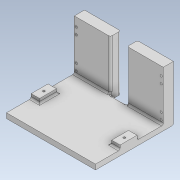
# Autodesk Inventor part: electrical_system_fix_board
Saved by Autodesk Inventor 2020 (Build 240168000, 168)
## iProperties
Created: 2021-01-08
Part Number: electrical_system_fix_board
Material: Generic
Document SubType Name: Modeling
Designer: DELL
Density: 1 g/cm^3
Appearance: Default
Author: DELL
Autodesk Inventor part; units mm, degrees
ref_plane "YZ Plane" through (0, 0, 0) normal (1, 0, 0) x (0, 1, 0)
ref_plane "XZ Plane" through (0, 0, 0) normal (0, 1, 0) x (-1, 0, 0)
ref_plane "XY Plane" through (0, 0, 0) normal (0, 0, 1) x (1, 0, 0)
sketch "Sketch1" plane through (0, 0, 0) normal (0, 0, 1) x (1, 0, 0)
  line L0 (52.5, 32.5) -> (-52.5, 32.5)
  line L1 (-52.5, 32.5) -> (-52.5, -32.5)
  line L2 (-52.5, -32.5) -> (52.5, -32.5)
  line L3 (52.5, -32.5) -> (52.5, 32.5)
  line L4 (52.5, 32.5) -> (-52.5, -32.5) construction
  line L5 (-52.5, 32.5) -> (52.5, -32.5) construction
  line L6 (-10, -32.5) -> (-52.5, -32.5)
  line L7 (-52.5, -32.5) -> (-52.5, 32.5)
  line L8 (-52.5, 32.5) -> (-10, 32.5)
  line L9 (-10, 32.5) -> (-10, -32.5)
  line L10 (-10, -32.5) -> (-52.5, 32.5) construction
  line L11 (-52.5, -32.5) -> (-10, 32.5) construction
  line L12 (10, -32.5) -> (52.5, -32.5)
  line L13 (52.5, -32.5) -> (52.5, 32.5)
  line L14 (52.5, 32.5) -> (10, 32.5)
  line L15 (10, 32.5) -> (10, -32.5)
  line L16 (10, -32.5) -> (52.5, 32.5) construction
  line L17 (52.5, -32.5) -> (10, 32.5) construction
  line L18 (0, 32.5) -> (0, -32.5) construction
  point P0 (0, 0)
  point P1 (-31.25, 0)
  point P2 (31.25, 0)
  point P3 (10, 32.5)
  point P4 (10, -32.5)
  point P5 (-10, 32.5)
  dimension "d0" = 105
  dimension "d1" = 65
  dimension "d2" = 20
  constraints: 38 end point, 8 midpoint, 6 parallel, 3 horizontal, 3 perpendicular, 2 collinear, 1 other
  measures "d0" distance between parallel lines of L3 L1
  measures "d1" distance between parallel lines of L2 L0
  measures "d2" distance between parallel lines of L15 L9
extrude "Extrusion1" add sketch "Sketch1" along normal blind 12 contours L3 L2 L15 L0 | L9 L2 L1 L0
sketch "Sketch2" plane through (0, 0, 12) normal (0, 0, 1) x (1, 0, 0)
  line L0 (-52.5, -32.5) -> (-10, -32.5) projected
  line L1 (52.5, -26.5) -> (-52.5, -26.5)
  line L2 (-52.5, -26.5) -> (-52.5, -32.5)
  line L3 (-52.5, -32.5) -> (52.5, -32.5)
  line L4 (52.5, -32.5) -> (52.5, -26.5)
  line L5 (52.5, -26.5) -> (-52.5, -32.5) construction
  line L6 (-52.5, -26.5) -> (52.5, -32.5) construction
  line L7 (52.5, -32.5) -> (52.5, 32.5) projected
  line L8 (42.5, -32.5) -> (-42.5, -32.5)
  line L9 (-42.5, -32.5) -> (-42.5, -26.5)
  line L10 (-42.5, -26.5) -> (42.5, -26.5)
  line L11 (42.5, -26.5) -> (42.5, -32.5)
  line L12 (42.5, -32.5) -> (-42.5, -26.5) construction
  line L13 (-42.5, -32.5) -> (42.5, -26.5) construction
  point P0 (0, 0)
  point P1 (0, -29.5)
  dimension "d5" = 6
  dimension "d31" = 85
  constraints: 24 end point, 4 midpoint, 4 parallel, 2 horizontal, 2 perpendicular, 1 collinear, 1 point on line
  measures "d5" distance between parallel lines of L3 L1
  measures "d31" distance between parallel lines of L11 L9
extrude "Extrusion2" add sketch "Sketch2" along normal blind 80
sketch "Sketch4" plane through (0, 0, 0) normal (0, 0, -1) x (-1, 0, 0)
  line L0 (-50, -22.5) -> (50, -22.5) construction
  line L1 (50, -22.5) -> (50, 22.5) construction
  line L2 (50, 22.5) -> (-50, 22.5) construction
  line L3 (-50, 22.5) -> (-50, -22.5) construction
  line L4 (-50, -22.5) -> (50, 22.5) construction
  line L5 (50, -22.5) -> (-50, 22.5) construction
  circle A0 centre (50, 22.5) radius 1.25
  circle A1 centre (-50, 22.5) radius 1.25
  circle A2 centre (-50, -22.5) radius 1.25
  circle A3 centre (50, -22.5) radius 1.25
  circle A4 centre (50, -14.5) radius 1.25
  circle A5 centre (50, -6.5) radius 1.25
  circle A6 centre (42, -22.5) radius 1.25
  line L6 (50, 0) -> (-50, 0) construction
  line L7 (0, -22.5) -> (0, 22.5) construction
  circle A7 centre (50, 22.5) radius 1.25
  circle A8 centre (50, 14.5) radius 1.25
  circle A9 centre (50, 6.5) radius 1.25
  circle A10 centre (42, 22.5) radius 1.25
  circle A11 centre (-50, -14.5) radius 1.25
  circle A12 centre (-50, -6.5) radius 1.25
  circle A13 centre (-42, -22.5) radius 1.25
  circle A14 centre (-42, 22.5) radius 1.25
  circle A15 centre (-50, 14.5) radius 1.25
  circle A16 centre (-50, 6.5) radius 1.25
  point P0 (0, 0)
  dimension "d13" = 100
  dimension "d14" = 45
  dimension "d16" = 2.5
  dimension "d35" = 8
  dimension "d36" = 8
  dimension "d37" = 8
  constraints: 17 centre point, 16 end point, 10 symmetric about line, 6 equal radius, 6 midpoint, 4 coincident, 3 point on line, 2 parallel, 1 horizontal, 1 perpendicular, 10 other
  measures "d13" distance of L1.end L2.end
  measures "d14" distance of L0.end L1.end
  measures "d16" diameter of A0
  measures "d35" distance of A4.centre L0.end
  measures "d36" distance of A4.centre A5.centre
  measures "d37" distance of L0.end A6.centre
extrude "Extrusion4" cut sketch "Sketch4" against normal through all contours A0 | A1 | A2 | A3 | A4 | A8 | A11 | A15
fillet "Fillet1" radius 2 2 edges at (-31.25, -26.5, 12) (31.25, -26.5, 12)
fillet "Fillet2" radius 2 11 edges at (10, -29.5, 12) (-10, -29.5, 12) (0, -26.5, 12) (-10, -25.9142, 12.5858) (-10, 4, 12) (10, -25.9142, 12.5858) (10, 4, 12) (10, 0, 0) (-10, 0, 0) (31.25, -32.5, 0) (-31.25, -32.5, 0)
sketch "Sketch6" plane through (-52.5, -26.5, 92) normal (0, 1, 0) x (1, 0, 0)
  line L0 (0, 78) -> (0, 0) construction
  line L1 (0, 39) -> (105, 39) construction
  line L2 (105, 90) -> (105, 0) construction
  circle A0 centre (5, 39) radius 1.25
  circle A1 centre (100, 39) radius 1.25
  line L3 (44.5, 80) -> (60.5, 80) construction
  line L4 (52.5, 80) -> (52.5, 0) construction
  line L5 (105, 0) -> (0, 0) construction
  line L6 (10, 49) -> (0, 49)
  line L7 (0, 49) -> (0, 29)
  line L8 (0, 29) -> (10, 29)
  line L9 (10, 29) -> (10, 49)
  line L10 (10, 49) -> (0, 29) construction
  line L11 (0, 49) -> (10, 29) construction
  line L12 (105, 78) -> (105, 0) projected
  line L13 (95, 29) -> (105, 29)
  line L14 (105, 29) -> (105, 49)
  line L15 (105, 49) -> (95, 49)
  line L16 (95, 49) -> (95, 29)
  line L17 (95, 29) -> (105, 49) construction
  line L18 (105, 29) -> (95, 49) construction
  point P0 (52.5, 92)
  dimension "d43" = 2.5
  dimension "d44" = 95
  dimension "d50" = 20
  constraints: 28 end point, 7 midpoint, 5 point on line, 4 parallel, 3 horizontal, 2 centre point, 2 perpendicular, 1 collinear, 1 equal radius, 1 symmetric about line
  measures "d43" diameter of A0
  measures "d44" distance of A1.centre A0.centre
  measures "d50" distance of L8.end L6.start
extrude "Extrusion8" cut sketch "Sketch6" against normal through all contours A0 | A1
extrude "Extrusion9" add sketch "Sketch6" along normal blind 5
fillet "Fillet3" radius 2 6 edges at (-47.5, -26.5, 63) (-42.5, -26.5, 53) (-47.5, -26.5, 43) (47.5, -26.5, 63) (42.5, -26.5, 53) (47.5, -26.5, 43)
equation "\"d36\" = d35"
equation "\"d37\" = d35"
body "Solid1"
